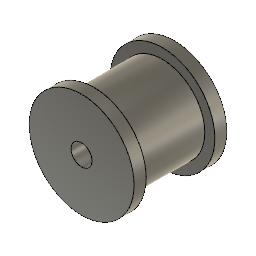
ROS_Tire_NonMotor (Autodesk Fusion 360 design; units mm, degrees)
Autodesk Fusion 360 part; units mm, degrees
sketch "Sketch1" plane through (0, 0, 0) normal (0, 1, 0) x (1, 0, 0)
  circle A0 centre (0, 0) radius 10.5
  dimension "d1" = 21
  constraint coincident A0.centre origin
  measures "d1" diameter of A0
extrude "Extrude1" add sketch "Sketch1" along normal blind 17
sketch "Sketch2" plane through (0, 0, 0) normal (0, -1, 0) x (1, 0, 0)
  circle A0 centre (0, 0) radius 10.5
  circle A1 centre (0, 0) radius 13
  dimension "d4" = 26
  constraint concentric A0 A1
  measures "d4" diameter of A1
extrude "Extrude2" add sketch "Sketch2" along normal blind 3 contours A0 | A1
sketch "Sketch3" plane through (0, 17, 0) normal (0, 1, 0) x (-1, 0, 0)
  circle A0 centre (0, 0) radius 10.5
  circle A1 centre (0, 0) radius 13
  dimension "d7" = 26
  constraint concentric A0 A1
  measures "d7" diameter of A1
extrude "Extrude3" add sketch "Sketch3" along normal blind 3 contours A0 | A1
sketch "Sketch4" plane through (0, -3, 0) normal (0, -1, 0) x (1, 0, 0)
  circle A0 centre (0, 0) radius 13
  circle A1 centre (0, 0) radius 2.6
  dimension "d10" = 5.2
  constraint coincident A0.centre A1.centre
  measures "d10" diameter of A1
extrude "Extrude4" cut sketch "Sketch4" against normal blind 6 contours A1
extrude "Extrude5" cut sketch "Sketch4" against normal blind 23 contours A1
